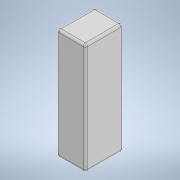
# Autodesk Inventor part: DikkeBatterij
Saved by Autodesk Inventor 2022 (Build 260153000, 153)
## iProperties
Created: 2022-03-24
Part Number: DikkeBatterij
Material: Generic
Document SubType Name: Modeling
Designer: 32497
Density: 1 g/cm^3
Appearance: Default
Author: 32497
Autodesk Inventor part; units mm, degrees
ref_plane "YZ Plane" through (0, 0, 0) normal (1, 0, 0) x (0, 1, 0)
ref_plane "XZ Plane" through (0, 0, 0) normal (0, 1, 0) x (-1, 0, 0)
ref_plane "XY Plane" through (0, 0, 0) normal (0, 0, 1) x (1, 0, 0)
sketch "Sketch1" plane through (0, 0, 0) normal (0, 1, 0) x (-1, 0, 0)
  line L0 (-13.1992, 17.25) -> (12.7008, 17.25)
  line L1 (12.7008, 17.25) -> (12.7008, -17.15)
  line L2 (12.7008, -17.15) -> (-13.1992, -17.15)
  line L3 (-13.1992, -17.15) -> (-13.1992, 17.25)
  line L4 (-13.1992, 17.25) -> (12.7008, -17.15) construction
  line L5 (12.7008, 17.25) -> (-13.1992, -17.15) construction
  point P0 (0, 0)
  point P1 (-0.2492, 0.05)
  dimension "d0" = 25.9
  dimension "d1" = 34.4
  constraints: 12 end point, 2 midpoint, 2 parallel, 1 horizontal, 1 perpendicular
  measures "d0" distance of L1.end L2.end
  measures "d1" distance of L0.end L1.end
extrude "Extrusion1" add sketch "Sketch1" along normal blind 100.4
fillet "Fillet1" radius 2 12 edges at (13.1992, 100.4, 0.05) (0.2492, 100.4, 17.25) (-12.7008, 100.4, 0.05) (0.2492, 100.4, -17.15) (13.1992, 0, 0.05) (0.2492, 0, 17.25) (-12.7008, 0, 0.05) (0.2492, 0, -17.15) (13.1992, 50.2, -17.15) (-12.7008, 50.2, -17.15) (13.1992, 50.2, 17.25) (-12.7008, 50.2, 17.25)
body "Solid1"
